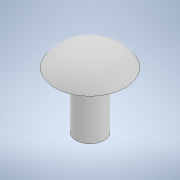
# Autodesk Inventor part: DERKS Linkage Peg
Saved by Autodesk Inventor 2020 (Build 240168000, 168)
## iProperties
Created: 2020-04-30
Part Number: DERKS Linkage Peg
Material: Generic
Document SubType Name: Modeling
Designer: tader
Density: 1 g/cm^3
Appearance: Default
Author: tader
Autodesk Inventor part; units mm, degrees
ref_plane "YZ Plane" through (0, 0, 0) normal (1, 0, 0) x (0, 1, 0)
ref_plane "XZ Plane" through (0, 0, 0) normal (0, 1, 0) x (-1, 0, 0)
ref_plane "XY Plane" through (0, 0, 0) normal (0, 0, 1) x (1, 0, 0)
sketch "Sketch1" plane through (0, 0, 0) normal (0, 0, 1) x (1, 0, 0)
  line L0 (-0.8768, 4.1275) -> (-0.8768, -4.1275)
  line L1 (-0.8768, -4.1275) -> (0.7107, -4.1275)
  line L2 (0.7107, -4.1275) -> (0.7107, 2.2225)
  line L3 (0.7107, 2.2225) -> (3.0907, 2.2225)
  arc A0 (3.0907, 2.2225) -> (-0.8768, 4.1275) centre (-0.322, 0.199) ccw
  point P0 (0, 0)
  dimension "d0" = 8.255
  dimension "d1" = 6.35
  dimension "d2" = 3.9675
  dimension "d3" = 3.9675
  dimension "d4" = 1.5875
  constraints: 8 end point, 3 perpendicular, 2 point on circle, 1 centre point, 1 vertical
  measures "d0" distance of L0.start L0.end
  measures "d1" distance between parallel lines of L1 L3
  measures "d2" distance from line of L3.end L0
  measures "d3" radius of A0
  measures "d4" distance of L1.end L0.end
revolve "Revolution1" add sketch "Sketch1" angle 360 about axis through (-0.8768, 4.1275, 0) along (0, -1, 0)
body "Solid1"
